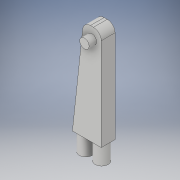
# Autodesk Inventor part: Forearm
Saved by Autodesk Inventor 2017 (Build 210142000, 142)
## iProperties
Created: 2017-05-25
Part Number: Forearm
Material: Generic
Document SubType Name: Modeling
Designer: garre
Density: 1 g/cm^3
Appearance: Default
Author: garre
Autodesk Inventor part; units mm, degrees
ref_plane "YZ Plane" through (0, 0, 0) normal (1, 0, 0) x (0, 1, 0)
ref_plane "XZ Plane" through (0, 0, 0) normal (0, 1, 0) x (-1, 0, 0)
ref_plane "XY Plane" through (0, 0, 0) normal (0, 0, 1) x (1, 0, 0)
sketch "Sketch1" plane through (0, 0, 0) normal (0, 0, 1) x (1, 0, 0)
  circle A0 centre (0, 0) radius 30.734
  line L0 (-56.515, -58.42) -> (56.515, -58.42)
  line L1 (56.515, -58.42) -> (56.515, 335.28)
  line L2 (56.515, 335.28) -> (-13.335, 335.28)
  line L3 (-13.335, 335.28) -> (-56.515, -58.42)
  dimension "d0" = 61.468
  dimension "d1" = 393.7
  dimension "d2" = 113.03
  dimension "d3" = 69.85
  dimension "d4" = 58.42
  dimension "d5" = 56.515
  constraints: 8 end point, 2 perpendicular, 1 centre point, 1 coincident, 1 horizontal
  measures "d0" diameter of A0
  measures "d1" distance of L0.end L1.end
  measures "d2" distance of L0.start L0.end
  measures "d3" distance of L1.end L2.end
  measures "d4" distance from line of L0 point (0, 0)
  measures "d5" distance from line of L1 point (0, 0)
extrude "Extrusion1" add sketch "Sketch1" against normal blind 54.3243
fillet "Fillet1" radius 30.48 2 edges at (56.515, 335.28, -27.1621) (-13.335, 335.28, -27.1621)
sketch "Sketch2" plane through (-56.515, -58.42, 0) normal (0, -1, 0) x (1, 0, 0)
  line L0 (113.03, 0) -> (113.03, -54.3243) projected
  line L1 (113.03, -27.1621) -> (0, -27.1621)
  line L2 (0, 0) -> (0, -54.3243) projected
  line L3 (56.515, -27.1621) -> (56.515, -44.3071)
  circle A0 centre (87.63, -27.1621) radius 25.4
  circle A1 centre (25.4, -27.1621) radius 25.4
  point P0 (56.515, 0)
  dimension "d10" = 50.8
  dimension "d9" = 50.8
  dimension "d11" = 113.03
  constraints: 4 end point, 3 midpoint, 2 point on line, 1 centre point, 1 horizontal alignment, 1 tangent, 1 vertical, 2 other
  measures "d9" diameter of A1
  measures "d11" distance of L1.start L1.end
extrude "Extrusion2" add sketch "Sketch2" along normal blind 71.12
sketch "Sketch3" plane through (0, 0, 0) normal (0, 0, 1) x (1, 0, 0)
  circle A0 centre (0, 0) radius 42.7153
  constraints: 1 centre point, 1 coincident
extrude "Extrusion3" add sketch "Sketch3" against normal blind 33.02
sketch "Sketch4" plane through (0, 0, -54.3243) normal (0, 0, -1) x (-1, 0, 0)
  line L0 (-26.035, 335.28) -> (-13.9848, 335.28) projected
  line L1 (-20.0099, 335.28) -> (-20.0099, 292.1)
  circle A0 centre (-20.0099, 292.1) radius 18.415
  point P0 (0, 0)
  dimension "d17" = 36.83
  dimension "d20" = 292.1
  constraints: 2 end point, 1 centre point, 1 coincident, 1 midpoint, 1 vertical
  measures "d17" diameter of A0
  measures "d20" vertical distance of point (0, 0) L1.end
extrude "Extrusion4" add sketch "Sketch4" against normal blind 83.82
equation "\"d5\" = 0.5 * d2"
equation "\"d10\" = d9"
body "Solid1"
